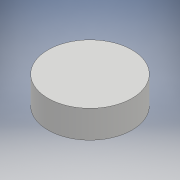
# Autodesk Inventor part: Roue
Saved by Autodesk Inventor 2017 SP1 (Build 210196100, 196)
## iProperties
Part Number: Roue
Material: Générique
Document SubType Name: Modeling
Designer: Sylvain
Density: 1 g/cm^3
Appearance: Par défaut
Author: Sylvain
Autodesk Inventor part; units mm, degrees
ref_plane "YZ Plane" through (0, 0, 0) normal (1, 0, 0) x (0, 1, 0)
ref_plane "XZ Plane" through (0, 0, 0) normal (0, 1, 0) x (-1, 0, 0)
ref_plane "XY Plane" through (0, 0, 0) normal (0, 0, 1) x (1, 0, 0)
sketch "Esquisse1" plane through (0, 0, 0) normal (0, 0, 1) x (1, 0, 0)
  circle A0 centre (0, 0) radius 15.2168
  dimension "d0" = 10
  constraints: 1 centre point, 1 coincident
extrude "Extrusion1" add sketch "Esquisse1" along normal blind 10
